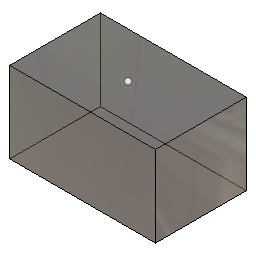
Slider Assembly FINAL v1 (Autodesk Fusion 360 archive; units mm, degrees)
design "Stock slider"
Autodesk Fusion 360 part; units mm, degrees
sketch "Sketch1" plane through (0, 0, 0) normal (0, 0, 1) x (1, 0, 0)
  line L0 (0, 0) -> (28.575, 0)
  line L1 (28.575, 0) -> (28.575, 17.78)
  line L2 (28.575, 17.78) -> (0, 17.78)
  line L3 (0, 17.78) -> (0, 0)
  dimension "d1" = 28.575
  dimension "d2" = 17.78
  constraint horizontal L0
  constraint vertical L1
  constraint horizontal L2
  constraint vertical L3
  constraint coincident L0.start L3.end
  measures "d1" distance of L1.end L2.end
  measures "d2" distance of L0.end L1.end
extrude "Extrude1" add sketch "Sketch1" along normal blind 15.875
sketch "Sketch2" plane through (0, 0, 15.875) normal (0, 0, 1) x (-1, 0, 0)
  line L0 (0, -17.78) -> (0, 0)
  line L1 (0, 0) -> (-28.575, 0)
  line L2 (-28.575, 0) -> (-28.575, -17.78)
  line L3 (-28.575, -17.78) -> (0, -17.78)
  point P0 (-14.2875, -8.89)
  dimension "d5" = 17.78
  dimension "d6" = 28.575
  dimension "d7" = 8.89
  dimension "d8" = 14.2875
  measures "d5" distance of L1.end L2.end
  measures "d6" distance of L0.start L2.end
  measures "d7" distance of L3 P0
  measures "d8" distance of L2 P0
equation "d7 = d5 / 2"
equation "d8 = d6 / 2"
